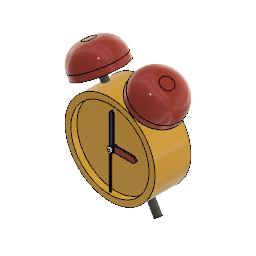
자명종 (Autodesk Fusion 360 design; units mm, degrees)
Autodesk Fusion 360 part; units mm, degrees
sketch "스케치1" plane through (0, 0, 0) normal (0, 1, 0) x (1, 0, 0)
  circle A0 centre (0, 0) radius 75
  dimension "d1" = 150
  constraint coincident A0.centre origin
  measures "d1" diameter of A0
extrude "돌출1" add sketch "스케치1" along normal mid plane 60 makes body 1
sketch "스케치2" plane through (0, -30, 0) normal (0, -1, 0) x (1, 0, 0)
  circle A0 centre (0, 0) radius 75
  circle A1 centre (0, 0) radius 65
  dimension "d4" = 130
  constraint concentric A0 A1
  measures "d4" diameter of A1
extrude "돌출2" cut sketch "스케치2" against normal blind 10 contours A1 bodies 1
sketch "스케치3" plane through (0, 0, 0) normal (0, 1, 0) x (1, 0, 0)
  line L0 (0, 100) -> (6, 100)
  line L1 (6, 100) -> (6, -90)
  line L2 (6, -90) -> (40, -90)
  line L3 (40, -90) -> (40, -130)
  line L4 (40, -130) -> (0, -130)
  line L5 (0, -130) -> (0, 100)
  dimension "d7" = 6
  dimension "d8" = 40
  dimension "d9" = 40
  dimension "d10" = 90
  dimension "d11" = 100
  constraint horizontal L0
  constraint perpendicular L0 L1
  constraint perpendicular L1 L2
  constraint perpendicular L2 L3
  constraint perpendicular L1 L4
  constraint perpendicular L0 L5
  constraint coincident origin L5
  measures "d7" distance of L0.start L0.end
  measures "d8" distance of L3.end L4.end
  measures "d9" distance of L2.end L3.end
  measures "d10" distance of origin L2
  measures "d11" distance of origin L0
revolve "회전1" add sketch "스케치3" angle 360 about axis through (0, 0, 130) along (0, 0, -1) separate body makes body 2
fillet "모깎기1" radius 30 1 edges at (-37.2931, -14.4646, 130) on bodies 2
move_body "이동1" bodies 2 to x (0.866025, 0, -0.5) y (0, 1, 0) z (0.5, 0, 0.866025) at (0, 0, 0)
mirror "미러1" about plane through (0, 0, 0) normal (1, 0, 0) of bodies 2 merged
sketch "스케치4" plane through (0, -20, 0) normal (0, -1, 0) x (1, 0, 0)
  circle A0 centre (0, 0) radius 65
  circle A1 centre (0, 0) radius 2.5
  dimension "d17" = 5
  constraint concentric A0 A1
  measures "d17" diameter of A1
extrude "돌출3" add sketch "스케치4" along normal blind 4 contours A1 bodies 1
sketch "스케치5" plane through (0, -24, 0) normal (0, -1, 0) x (1, 0, 0)
  circle A0 centre (0, 0) radius 2.5
  line L0 (-5, 5) -> (40, 5)
  line L1 (40, 5) -> (40, -5)
  line L2 (40, -5) -> (-5, -5)
  line L3 (-5, -5) -> (-5, 5)
  dimension "d20" = 45
  dimension "d21" = 10
  dimension "d22" = 5
  dimension "d23" = 5
  constraint horizontal L0
  constraint vertical L1
  constraint horizontal L2
  constraint vertical L3
  measures "d20" distance of L1 L3
  measures "d21" distance of L0.start L2.end
  measures "d22" distance of A0.centre L3
  measures "d23" distance of A0.centre L0
extrude "돌출4" add sketch "스케치5" along normal blind 2 separate body makes body 3
chamfer "모따기1" distance 5 angle 45 2 edges at (40, -25, 5) (40, -25, -5) on bodies 3
sketch "스케치6" plane through (0, -26, 0) normal (0, -1, 0) x (1, 0, 0)
  circle A0 centre (0, 0) radius 2.5
  line L0 (35, -5) -> (40, 0)
  line L1 (40, 0) -> (35, 5)
  line L2 (35, 5) -> (-5, 5)
  line L3 (-5, 5) -> (-5, -5)
  line L4 (-5, -5) -> (35, -5)
  line L5 (-3, 55) -> (3, 55)
  line L6 (3, 55) -> (3, -5)
  line L7 (3, -5) -> (-3, -5)
  line L8 (-3, -5) -> (-3, 55)
  dimension "d27" = 60
  dimension "d28" = 6
  dimension "d29" = 3
  constraint horizontal L5
  constraint vertical L6
  constraint horizontal L7
  constraint vertical L8
  constraint collinear L4 L7
  measures "d27" distance of L5.start L7.end
  measures "d28" distance of L5.start L5.end
  measures "d29" distance of A0.centre L8
extrude "돌출5" add sketch "스케치6" along normal blind 2 separate body contours L2 L4 L6 L7 L8 | L2 L5 L6 L8 makes body 4
chamfer "모따기2" distance 3 angle 45 2 edges at (-3, -27, 55) (3, -27, 55) on bodies 4
sketch "스케치7" plane through (0, -28, 0) normal (0, -1, 0) x (1, 0, 0)
  circle A0 centre (0, 0) radius 2.5
  line L0 (3, 52) -> (0, 55)
  line L1 (0, 55) -> (-3, 52)
  line L2 (-3, 52) -> (-3, -5)
  line L3 (-3, -5) -> (3, -5)
  line L4 (3, -5) -> (3, 52)
  circle A1 centre (0, 0) radius 4.5
  line L5 (-1, -1.5) -> (1, -1.5)
  line L6 (1, -1.5) -> (1, -61.5)
  line L7 (1, -61.5) -> (-1, -61.5)
  line L8 (-1, -61.5) -> (-1, -1.5)
  dimension "d33" = 9
  dimension "d34" = 2
  dimension "d35" = 60
  dimension "d36" = 1.5
  dimension "d37" = 1
  constraint concentric A0 A1
  constraint horizontal L5
  constraint vertical L6
  constraint horizontal L7
  constraint vertical L8
  measures "d33" diameter of A1
  measures "d34" distance of L5.start L5.end
  measures "d35" distance of L5.start L7.end
  measures "d36" distance of A0.centre L5
  measures "d37" distance of A0.centre L8
extrude "돌출6" add sketch "스케치7" along normal blind 2 contours A0 L2 L4 A1 L6 L8 | A0 A1 L6 L8 | L3 A1 L6 L8 | L2 A1 | L3 L6 L7 L8 | L4 A1 bodies 4
extrude "돌출7" add 1 faces at (-0.8863, -24, 0.2321) along direction (0, -1, 0) up to surface (6 mm away) separate body on bodies 1 makes body 5
sketch "스케치8" plane through (0, -30, 0) normal (0, -1, 0) x (1, 0, 0)
  circle A0 centre (0, 0) radius 2.5
  arc A1 (1, -4.3875) -> (-1, -4.3875) centre (0, 0) ccw
  line L0 (-1, -4.3875) -> (-1, -61.5)
  line L1 (-1, -61.5) -> (1, -61.5)
  line L2 (1, -61.5) -> (1, -4.3875)
  circle A2 centre (0, 0) radius 4
  dimension "d42" = 8
  constraint coincident A0.centre A1.centre
  measures "d42" diameter of A2
extrude "돌출8" add sketch "스케치8" along normal blind 2 contours A0 | A2 bodies 5
fillet "모깎기2" radius 2 1 edges at (-3.7293, -32, -1.4465) on bodies 5
sketch "스케치9" plane through (0, 0, -5) normal (0, 0, -1) x (1, 0, 0)
  line L0 (-3, 26) -> (3, 26)
  line L1 (3, 26) -> (3, 28)
  line L2 (3, 28) -> (1, 28)
  line L3 (1, 28) -> (-1, 28)
  line L4 (-1, 28) -> (-3, 28)
  line L5 (-3, 28) -> (-3, 26)
  line L6 (3, 26) -> (-3, 26)
  line L7 (-3, 26) -> (-3, 28)
  line L8 (-3, 28) -> (3, 28)
  line L9 (3, 28) -> (3, 26)
  dimension "d47" = 6
  dimension "d48" = 2
  constraint horizontal L6
  constraint vertical L7
  constraint horizontal L8
  constraint vertical L9
  constraint coincident L0.end L1.start
  measures "d47" distance of L0.end L0.start
  measures "d48" distance of L0.end L1.end
split "분할1" by curves path "스케치9" along L7 L8 L9 L6 bodies 4 makes body 6 at (-0.3333, -30, -23.425)
